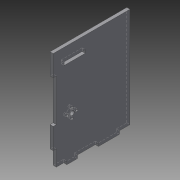
# Autodesk Inventor part: Motor support
Saved by Autodesk Inventor 2015 (Build 190159000, 159)
## iProperties
Created: 2014-11-11
Part Number: Motor support
Material: Generic
Document SubType Name: Modeling
Designer: karl
Density: 1 g/cm^3
Appearance: Default
Author: karl
Autodesk Inventor part; units mm, degrees
ref_plane "YZ Plane" through (0, 0, 0) normal (1, 0, 0) x (0, 1, 0)
ref_plane "XZ Plane" through (0, 0, 0) normal (0, 1, 0) x (-1, 0, 0)
ref_plane "XY Plane" through (0, 0, 0) normal (0, 0, 1) x (1, 0, 0)
sketch "Sketch1" plane through (0, 0, 0) normal (1, 0, 0) x (0, 1, 0)
  line L0 (-35, -47.5) -> (35, -47.5)
  line L1 (35, -47.5) -> (35, 47.5)
  line L2 (35, 47.5) -> (-35, 47.5)
  line L3 (-35, 47.5) -> (-35, -47.5)
  line L4 (-35, -47.5) -> (35, 47.5) construction
  line L5 (35, -47.5) -> (-35, 47.5) construction
  point P0 (0, 0)
  dimension "d0" = 70
  dimension "d1" = 95
  constraints: 12 end point, 2 midpoint, 2 parallel, 1 horizontal, 1 perpendicular
  measures "d0" distance of L2.end L1.end
  measures "d1" distance of L1.end L0.end
extrude "Extrusion1" add sketch "Sketch1" along normal blind 3
sketch "Sketch2" plane through (3, 0, 0) normal (1, 0, 0) x (0, 0, -1)
  line L0 (-47.5, -35) -> (47.5, -35) projected
  line L1 (32.5, -35) -> (12.5, -35)
  line L2 (12.5, -35) -> (12.5, -38)
  line L3 (12.5, -38) -> (32.5, -38)
  line L4 (32.5, -38) -> (32.5, -35)
  line L5 (-27.5, -35) -> (-47.5, -35)
  line L6 (-47.5, -35) -> (-47.5, -38)
  line L7 (-47.5, -38) -> (-27.5, -38)
  line L8 (-27.5, -38) -> (-27.5, -35)
  line L9 (47.5, -35) -> (47.5, 35) projected
  point P0 (0, 0)
  dimension "d4" = 20
  dimension "d5" = 3
  dimension "d6" = 20
  dimension "d7" = 3
  dimension "d8" = 40
  dimension "d9" = 15
  constraints: 16 end point, 4 parallel, 2 horizontal, 2 perpendicular, 2 point on line
  measures "d4" distance of L3.end L2.end
  measures "d5" distance of L2.end L1.end
  measures "d6" distance of L7.end L6.end
  measures "d7" distance of L6.end L5.end
  measures "d8" distance between parallel lines of L2 L8
  measures "d9" distance between parallel lines of L9 L4
extrude "Extrusion2" add sketch "Sketch2" against normal blind 3
sketch "Sketch3" plane through (3, 0, 0) normal (1, 0, 0) x (0, 0, -1)
  line L0 (47.5, -35) -> (47.5, 35) projected
  line L1 (47.5, 25) -> (50.5, 25)
  line L2 (50.5, 25) -> (50.5, 5)
  line L3 (50.5, 5) -> (47.5, 5)
  line L4 (47.5, 5) -> (47.5, 25)
  line L5 (47.5, 35) -> (-47.5, 35) projected
  line L6 (47.5, -15) -> (50.5, -15)
  line L7 (50.5, -15) -> (50.5, -25)
  line L8 (50.5, -25) -> (47.5, -25)
  line L9 (47.5, -25) -> (47.5, -15)
  line L10 (32.5, -35) -> (47.5, -35) projected
  point P0 (0, 0)
  dimension "d12" = 3
  dimension "d13" = 20
  dimension "d14" = 10
  dimension "d15" = 3
  dimension "d16" = 10
  dimension "d17" = 10
  dimension "d18" = 20
  constraints: 16 end point, 4 parallel, 2 horizontal, 2 perpendicular, 2 point on line
  measures "d12" distance of L2.end L3.end
  measures "d13" distance of L1.end L2.end
  measures "d14" distance between parallel lines of L5 L1
  measures "d15" distance of L7.end L8.end
  measures "d16" distance of L6.end L7.end
  measures "d17" distance between parallel lines of L10 L8
  measures "d18" distance between parallel lines of L3 L6
extrude "Extrusion3" add sketch "Sketch3" against normal blind 3
sketch "Sketch4" plane through (3, 0, 0) normal (1, 0, 0) x (0, 0, -1)
  line L0 (32.5, -35) -> (32.5, -38) projected
  line L1 (40.5, -38) -> (32.5, -38) projected
  line L2 (40.5, -35) -> (40.5, -38) projected
  line L3 (32.5, -35) -> (40.5, -35) projected
  line L4 (12.5, -38) -> (12.5, -35) projected
  line L5 (-19.5, -35) -> (12.5, -35) projected
  line L6 (-19.5, -35) -> (-19.5, -38) projected
  line L7 (12.5, -38) -> (-19.5, -38) projected
  circle A0 centre (10.5, -20) radius 30 construction
  circle A1 centre (10.5, -20) radius 2
  point P0 (0, 0)
  dimension "d21" = 60
  dimension "d22" = 30
  dimension "d23" = 15
  dimension "d24" = 4
  constraints: 2 centre point, 1 coincident
  measures "d21" diameter of A0
  measures "d22" distance from line of A0.centre L2
  measures "d23" distance from line of L5 A0.centre
  measures "d24" diameter of A1
extrude "Extrusion4" cut sketch "Sketch4" against normal blind 3 contours A1
sketch "Sketch5" plane through (3, 0, 0) normal (1, 0, 0) x (0, 0, -1)
  circle A0 centre (10.5, -15.5) radius 1
  circle A1 centre (10.5, -20) radius 2 projected
  circle A2 centre (6, -20) radius 1
  circle A3 centre (10.5, -24.5) radius 1
  circle A4 centre (15, -20) radius 1
  point P0 (0, 0)
  dimension "d27" = 2
  dimension "d28" = 4.5
  dimension "d31" = 360
  constraints: 4 centre point, 1 vertical alignment, 9 other
  measures "d27" diameter of A0
  measures "d28" distance of A1.centre A0.centre
extrude "Extrusion5" cut sketch "Sketch5" against normal blind 3 contours A0 | A2 | A3 | A4
sketch "Sketch6" plane through (0, 0, 0) normal (-1, 0, 0) x (0, 0, 1)
  line L0 (32.5, -7.5) -> (35.5, -7.5)
  line L1 (35.5, -7.5) -> (35.5, -27.5)
  line L2 (35.5, -27.5) -> (32.5, -27.5)
  line L3 (32.5, -27.5) -> (32.5, -7.5)
  line L4 (-47.5, -15) -> (-47.5, 5) projected
  line L5 (27.5, -35) -> (-12.5, -35) projected
  point P0 (0, 0)
  dimension "d35" = 3
  dimension "d36" = 20
  dimension "d37" = 80
  dimension "d38" = 7.5
  constraints: 8 end point, 2 parallel, 1 horizontal, 1 perpendicular
  measures "d35" distance of L1.end L2.end
  measures "d36" distance of L0.end L1.end
  measures "d37" distance between parallel lines of L4 L3
  measures "d38" distance between parallel lines of L5 L2
extrude "Extrusion6" cut sketch "Sketch6" against normal blind 10
sketch "Sketch7" plane through (0, 0, 0) normal (-1, 0, 0) x (0, 0, 1)
  line L0 (-32.5, 3) -> (-12.5, 3)
  line L1 (-12.5, 3) -> (-12.5, 0)
  line L2 (-12.5, 0) -> (-32.5, 0)
  line L3 (-32.5, 0) -> (-32.5, 3)
  line L4 (27.5, -35) -> (-12.5, -35) projected
  line L5 (-47.5, -15) -> (-47.5, 5) projected
  line L6 (17.5, 3) -> (37.5, 3)
  line L7 (37.5, 3) -> (37.5, 0)
  line L8 (37.5, 0) -> (17.5, 0)
  line L9 (17.5, 0) -> (17.5, 3)
  point P0 (0, 0)
  dimension "d41" = 20
  dimension "d42" = 3
  dimension "d43" = 35
  dimension "d44" = 15
  dimension "d45" = 20
  dimension "d46" = 3
  dimension "d47" = 30
  constraints: 16 end point, 4 parallel, 2 horizontal, 2 perpendicular, 1 collinear
  measures "d41" distance of L1.end L2.end
  measures "d42" distance of L0.end L1.end
  measures "d43" distance between parallel lines of L4 L2
  measures "d44" distance between parallel lines of L5 L3
  measures "d45" distance of L7.end L8.end
  measures "d46" distance of L6.end L7.end
  measures "d47" distance between parallel lines of L9 L1
extrude "Extrusion7" cut sketch "Sketch7" against normal blind 10
sketch "Sketch8" plane through (0, 0, 0) normal (-1, 0, 0) x (0, 0, 1)
  line L0 (-32.5, 23) -> (-29.5, 23)
  line L1 (-29.5, 23) -> (-29.5, 13)
  line L2 (-29.5, 13) -> (-32.5, 13)
  line L3 (-32.5, 13) -> (-32.5, 23)
  line L4 (18.5, 23) -> (15.5, 23)
  line L5 (15.5, 23) -> (15.5, 13)
  line L6 (15.5, 13) -> (18.5, 13)
  line L7 (18.5, 13) -> (18.5, 23)
  line L8 (-47.5, 25) -> (-47.5, 35) projected
  line L9 (-32.5, 3) -> (-12.5, 3) projected
  point P0 (0, 0)
  dimension "d50" = 3
  dimension "d51" = 10
  dimension "d52" = 3
  dimension "d53" = 10
  dimension "d54" = 15
  dimension "d55" = 45
  dimension "d56" = 10
  constraints: 16 end point, 4 parallel, 2 horizontal, 2 perpendicular, 1 point on line
  measures "d50" distance of L1.end L2.end
  measures "d51" distance of L0.end L1.end
  measures "d52" distance of L6.end L5.end
  measures "d53" distance of L5.end L4.end
  measures "d54" distance between parallel lines of L3 L8
  measures "d55" distance between parallel lines of L1 L5
  measures "d56" distance between parallel lines of L9 L2
extrude "Extrusion8" cut sketch "Sketch8" against normal blind 3
sketch "Sketch9" plane through (3, 0, 0) normal (1, 0, 0) x (0, 0, -1)
  line L0 (-35.5, 18) -> (-25.5, 18)
  line L1 (-25.5, 18) -> (-25.5, 15)
  line L2 (-25.5, 15) -> (-35.5, 15)
  line L3 (-35.5, 15) -> (-35.5, 18)
  line L4 (-37.5, 3) -> (-17.5, 3) projected
  line L5 (-18.5, 13) -> (-18.5, 23) projected
  point P0 (0, 0)
  dimension "d59" = 10
  dimension "d60" = 12
  dimension "d61" = 3
  dimension "d62" = 7
  constraints: 8 end point, 2 parallel, 1 horizontal, 1 perpendicular
  measures "d59" distance of L1.end L2.end
  measures "d60" distance between parallel lines of L2 L4
  measures "d61" distance between parallel lines of L2 L0
  measures "d62" distance between parallel lines of L5 L1
extrude "Extrusion9" cut sketch "Sketch9" against normal blind 3
sketch "Sketch10" plane through (0, 0, 0) normal (-1, 0, 0) x (0, 0, 1)
  line L0 (-47.5, 35) -> (47.5, 35) projected
  line L1 (-37.5, 35) -> (-17.5, 35)
  line L2 (-17.5, 35) -> (-17.5, 38)
  line L3 (-17.5, 38) -> (-37.5, 38)
  line L4 (-37.5, 38) -> (-37.5, 35)
  line L5 (22.5, 35) -> (42.5, 35)
  line L6 (42.5, 35) -> (42.5, 38)
  line L7 (42.5, 38) -> (22.5, 38)
  line L8 (22.5, 38) -> (22.5, 35)
  line L9 (-7.5, 35) -> (2.5, 35)
  line L10 (2.5, 35) -> (2.5, 38)
  line L11 (2.5, 38) -> (-7.5, 38)
  line L12 (-7.5, 38) -> (-7.5, 35)
  line L13 (-47.5, 25) -> (-47.5, 35) projected
  point P0 (0, 0)
  dimension "d65" = 20
  dimension "d66" = 3
  dimension "d67" = 20
  dimension "d68" = 3
  dimension "d69" = 10
  dimension "d70" = 3
  dimension "d71" = 10
  dimension "d72" = 10
  dimension "d73" = 20
  constraints: 24 end point, 6 parallel, 3 horizontal, 3 perpendicular, 3 point on line
  measures "d65" distance of L3.end L2.end
  measures "d66" distance of L2.end L1.end
  measures "d67" distance of L7.end L6.end
  measures "d68" distance of L6.end L5.end
  measures "d69" distance of L11.end L10.end
  measures "d70" distance of L10.end L9.end
  measures "d71" distance between parallel lines of L13 L4
  measures "d72" distance between parallel lines of L12 L2
  measures "d73" distance between parallel lines of L8 L10
extrude "Extrusion10" add sketch "Sketch10" against normal blind 3
sketch "Sketch11" plane through (0, 0, 0) normal (-1, 0, 0) x (0, 0, 1)
  line L0 (-47.5, -15) -> (-47.5, 5) projected
  line L1 (-47.5, 0) -> (-42.5, 0)
  line L2 (-42.5, 0) -> (-42.5, -3)
  line L3 (-42.5, -3) -> (-47.5, -3)
  line L4 (-47.5, -3) -> (-47.5, 0)
  line L5 (-12.5, 0) -> (-32.5, 0) projected
  point P0 (0, 0)
  dimension "d76" = 5
  dimension "d77" = 3
  constraints: 8 end point, 2 parallel, 1 collinear, 1 horizontal, 1 perpendicular, 1 point on line
  measures "d76" distance of L2.end L3.end
  measures "d77" distance of L1.end L2.end
extrude "Extrusion11" cut sketch "Sketch11" against normal blind 3
sketch "Sketch12" plane through (0, 0, 0) normal (-1, 0, 0) x (0, 0, 1)
  line L0 (47.5, 35) -> (47.5, -38) projected
  line L1 (47.5, 0) -> (42.5, 0)
  line L2 (42.5, 0) -> (42.5, -3)
  line L3 (42.5, -3) -> (47.5, -3)
  line L4 (47.5, -3) -> (47.5, 0)
  line L5 (37.5, 0) -> (17.5, 0) projected
  point P0 (0, 0)
  dimension "d80" = 3
  dimension "d81" = 5
  constraints: 8 end point, 2 parallel, 1 collinear, 1 horizontal, 1 perpendicular, 1 point on line
  measures "d80" distance of L1.end L2.end
  measures "d81" distance of L2.end L3.end
extrude "Extrusion12" cut sketch "Sketch12" against normal blind 3
body "Solid1"
